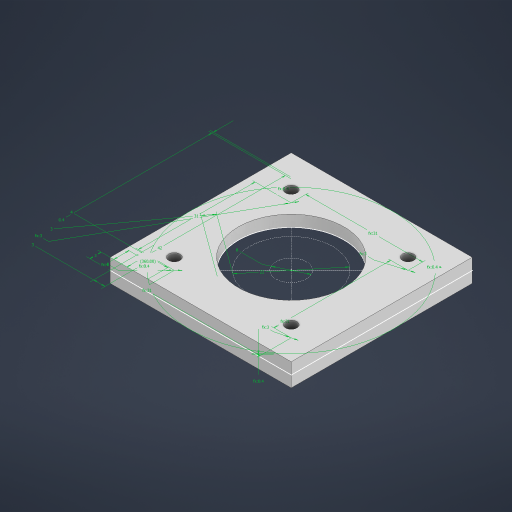
# Autodesk Inventor part: Stepper Holder
Saved by Autodesk Inventor 2024.2 (Build 282272000, 272)
## iProperties
Created: 2024-10-02
Part Number: Stepper Holder
Material: Generic
Document SubType Name: Modeling
Designer: jerem
Density: 1 g/cm^3
Appearance: Default
Author: jerem
Autodesk Inventor part; units mm, degrees
ref_plane "YZ Plane" through (0, 0, 0) normal (1, 0, 0) x (0, 1, 0)
ref_plane "XZ Plane" through (0, 0, 0) normal (0, 1, 0) x (-1, 0, 0)
ref_plane "XY Plane" through (0, 0, 0) normal (0, 0, 1) x (1, 0, 0)
sketch "Sketch1" plane through (0, 0, 0) normal (0, 1, 0) x (-1, 0, 0)
  line L0 (-21, -21) -> (21, -21) construction
  line L1 (21, -21) -> (21, 21) construction
  line L2 (21, 21) -> (-21, 21) construction
  line L3 (-21, 21) -> (-21, -21) construction
  line L4 (-21, -21) -> (21, 21) construction
  line L5 (21, -21) -> (-21, 21) construction
  circle A0 centre (15.5, 15.5) radius 1.5
  circle A1 centre (15.5, -15.5) radius 1.5
  circle A2 centre (-15.5, -15.5) radius 1.5
  circle A3 centre (-15.5, 15.5) radius 1.5
  circle A4 centre (0, 0) radius 11 construction
  circle A5 centre (0, 0) radius 4 construction
  circle A6 centre (0, 0) radius 14
  line L6 (-24, -24) -> (24, -24)
  line L7 (24, -24) -> (24, 24)
  line L8 (24, 24) -> (-24, 24)
  line L9 (-24, 24) -> (-24, -24)
  line L10 (-24, -24) -> (24, 24) construction
  line L11 (24, -24) -> (-24, 24) construction
  line L12 (21.4, -21.4) -> (-21.4, -21.4)
  line L13 (-21.4, -21.4) -> (-21.4, 21.4)
  line L14 (-21.4, 21.4) -> (21.4, 21.4)
  line L15 (21.4, 21.4) -> (21.4, -21.4)
  line L16 (21, 17) -> (17, 21) construction
  line L17 (-17, 21) -> (-21, 17) construction
  line L18 (-21, -17) -> (-17, -21) construction
  line L19 (17, -21) -> (21, -17) construction
  line L20 (17.1657, -21.4) -> (21.4, -17.1657)
  line L21 (-17.1657, -21.4) -> (-21.4, -17.1657)
  line L22 (-21.4, 17.1657) -> (-17.1657, 21.4)
  line L23 (17.1657, 21.4) -> (21.4, 17.1657)
  dimension "d0" = 42
  dimension "d1" = 31
  dimension "d2" = 31
  dimension "d3" = 31
  dimension "d4" = 31
  dimension "d5" = 3
  dimension "d6" = 3
  dimension "d7" = 3
  dimension "d8" = 3
  dimension "d9" = 22
  dimension "d10" = 8
  dimension "d12" = 3
  dimension "d13" = 3
  dimension "d14" = 3
  dimension "d17" = 0.4
  dimension "d20" = 4
  dimension "d21" = 4
  dimension "d24" = 360
  dimension "d26" = 0.4
  dimension "d27" = 0.4
  dimension "d28" = 0.4
  dimension "d29" = 0.4
  constraints: 48 end point, 17 point on line, 9 parallel, 7 centre point, 4 coincident, 4 midpoint, 4 perpendicular, 3 horizontal, 13 other
  measures "d0" distance of L0.end L1.end
  measures "d1" distance of A1.centre A0.centre
  measures "d2" distance of A2.centre A1.centre
  measures "d3" distance of A3.centre A2.centre
  measures "d4" distance of A0.centre A3.centre
  measures "d5" diameter of A0
  measures "d6" diameter of A1
  measures "d7" diameter of A2
  measures "d8" diameter of A3
  measures "d9" diameter of A4
  measures "d10" diameter of A5
  measures "d12" distance between parallel lines of L7 L1
  measures "d13" distance between parallel lines of L8 L2
  measures "d14" radial gap between concentric circles of A6 A4
  measures "d17" distance between parallel lines of L0 L12
  measures "d20" distance of L1.end L16.end
  measures "d21" distance of L1.end L16.start
  measures "d26" distance between parallel lines of L19 L20
  measures "d27" distance between parallel lines of L18 L21
  measures "d28" distance between parallel lines of L17 L22
  measures "d29" distance between parallel lines of L16 L23
extrude "Extrusion1" add sketch "Sketch1" along normal blind 3 contours L9 L8 L7 L6 | L12 L20 L15 | L12 L21 L13 L22 L14 L23 L15 L20 | L12 L13 L21 | L23 L14 L15 | L13 L14 L22
extrude "Extrusion2" add sketch "Sketch1" against normal blind 3 contours L9 L8 L7 L6
equation "\"d2\" = d1"
equation "\"d3\" = d1"
equation "\"d4\" = d1"
equation "\"d6\" = d5"
equation "\"d7\" = d5"
equation "\"d8\" = d5"
equation "\"d21\" = d20"
equation "\"d26\" = d17"
equation "\"d27\" = d17"
equation "\"d28\" = d17"
equation "\"d29\" = d17"
body "Solid1"
